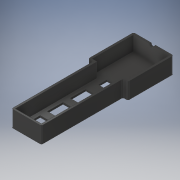
# Autodesk Inventor part: ajTop
Saved by Autodesk Inventor 2018 (Build 220112000, 112)
## iProperties
Created: 2018-02-03
Part Number: ajTop
Material: Generic
Document SubType Name: Modeling
Designer: Mom
Density: 1 g/cm^3
Appearance: Default
Author: Mom
Autodesk Inventor part; units mm, degrees
ref_plane "YZ Plane" through (0, 0, 0) normal (1, 0, 0) x (0, 1, 0)
ref_plane "XZ Plane" through (0, 0, 0) normal (0, 1, 0) x (-1, 0, 0)
ref_plane "XY Plane" through (0, 0, 0) normal (0, 0, 1) x (1, 0, 0)
sketch "Sketch1" plane through (0, 0, 0) normal (0, 1, 0) x (-1, 0, 0)
  line L0 (0, 0) -> (42, 0)
  line L1 (42, 0) -> (42, -115)
  line L2 (42, -115) -> (0, -115)
  line L3 (0, -115) -> (0, 0)
  line L4 (21, -115) -> (21, 0) construction
  line L5 (-7, -115) -> (49, -115)
  line L6 (49, -115) -> (49, -179)
  line L7 (49, -179) -> (-7, -179)
  line L8 (-7, -179) -> (-7, -115)
  line L9 (21, -179) -> (21, -115) construction
  dimension "d28" = 42
  dimension "d29" = 115
  dimension "d30" = 64
  dimension "d31" = 56
  constraints: 20 end point, 4 parallel, 3 midpoint, 2 collinear, 2 horizontal, 2 perpendicular
  measures "d28" distance of L1.end L2.end
  measures "d29" distance of L0.end L1.end
  measures "d30" distance of L5.end L6.end
  measures "d31" distance of L6.end L7.end
extrude "Extrusion1" add sketch "Sketch1" along normal blind 23
shell "Shell1" thickness 2.54 removed faces 1 at (-28, 23, -76.6667)
sketch "Sketch2" plane through (0, 0, 0) normal (0, -1, 0) x (1, 0, 0)
  line L0 (0, 0) -> (-42, 0) projected
  line L1 (-42, 0) -> (-42, -115) projected
  line L2 (0, -115) -> (0, 0) projected
  line L3 (-42, 0) -> (0, 0) projected
  line L4 (-21, 0) -> (-21, -111.5942) construction
  line L5 (-8, -10) -> (-34, -10)
  line L6 (-34, -10) -> (-34, -32.25)
  line L7 (-34, -32.25) -> (-8, -32.25)
  line L8 (-8, -32.25) -> (-8, -10)
  line L9 (-8, -42.25) -> (-34, -42.25)
  line L10 (-34, -42.25) -> (-34, -64.5)
  line L11 (-34, -64.5) -> (-8, -64.5)
  line L12 (-8, -64.5) -> (-8, -42.25)
  line L13 (-8, -74.5) -> (-34, -74.5)
  line L14 (-34, -74.5) -> (-34, -96.75)
  line L15 (-34, -96.75) -> (-8, -96.75)
  line L16 (-8, -96.75) -> (-8, -74.5)
  line L17 (-21, -10) -> (-21, -32.25) construction
  line L18 (-30.65, -110.75) -> (-11.35, -110.75)
  line L19 (-11.35, -110.75) -> (-11.35, -123.2)
  line L20 (-11.35, -123.2) -> (-30.65, -123.2)
  line L21 (-30.65, -123.2) -> (-30.65, -110.75)
  line L22 (-21, -123.2) -> (-21, -110.75) construction
  dimension "d33" = 10
  dimension "d34" = 10
  dimension "d35" = 26
  dimension "d36" = 22.25
  dimension "d37" = 10
  dimension "d46" = 12.45
  dimension "d47" = 19.3
  dimension "d48" = 14
  constraints: 38 end point, 8 parallel, 5 collinear, 5 midpoint, 4 horizontal, 4 perpendicular, 3 point on line, 1 vertical
  measures "d33" distance between parallel lines of L9 L7
  measures "d34" distance between parallel lines of L13 L11
  measures "d35" distance of L5.start L5.end
  measures "d36" distance of L7.end L5.start
  measures "d37" distance between parallel lines of L0 L5
  measures "d46" distance of L18.end L19.end
  measures "d47" distance of L18.start L18.end
  measures "d48" vertical distance of L18.start L14.end
extrude "Extrusion2" cut sketch "Sketch2" against normal blind 10
fillet "Fillet1" radius 2 8 edges at (0, 11.5, -115) (7, 11.5, -115) (0, 11.5, 0) (-42, 11.5, 0) (-42, 11.5, -115) (-49, 11.5, -115) (7, 11.5, -179) (-49, 11.5, -179)
sketch "Sketch3" plane through (5, 0, -179) normal (0, 0, -1) x (-1, 0, 0)
  line L0 (0, 23) -> (52, 23) projected
  line L1 (45, 23) -> (7, 23) projected
  line L2 (26, 23) -> (26, 16.6961) construction
  circle A0 centre (26, 23) radius 3.1
  line L3 (-2, 23) -> (-2, 0) projected
  line L4 (54, 0) -> (54, 23) projected
  point P0 (5, 0)
  dimension "d41" = 6.2
  dimension "d42" = 28
  dimension "d43" = 28
  constraints: 2 end point, 1 centre point, 1 coincident, 1 midpoint, 1 vertical
  measures "d41" diameter of A0
  measures "d42" distance from line of L3 L2.start
  measures "d43" distance from line of L4 L2.start
extrude "Extrusion3" cut sketch "Sketch3" against normal blind 10
equation "\"d33\" = d37"
equation "\"d34\" = d33"
body "Solid1"
